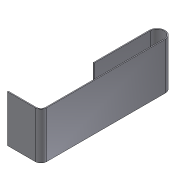
# Autodesk Inventor part: battery_tab_folded
Saved by Autodesk Inventor 2014 SP1 (Build 180222100, 222)
## iProperties
Created: 2013-03-29
Part Number: battery_tab_folded
Document SubType Name: Modeling
Designer: Robert Davis
Density: 7.85 g/cm^3
Material: Steel
Mass: 0.0909133 g
Surface Area: 2.37259 cm^2
Volume: 0.0115813 cm^3
Appearance: Steel
Author: Robert Davis
Autodesk Inventor part; units mm, degrees
ref_plane "YZ Plane" through (0, 0, 0) normal (1, 0, 0) x (0, 1, 0)
ref_plane "XZ Plane" through (0, 0, 0) normal (0, 1, 0) x (-1, 0, 0)
ref_plane "XY Plane" through (0, 0, 0) normal (0, 0, 1) x (1, 0, 0)
sketch "Sketch1" plane through (0, 0, 0) normal (0, 0, 1) x (1, 0, 0)
  line L0 (0, -3) -> (0, 3)
  line L1 (1.5, 3) -> (1.5, -9.7)
  line L2 (1, -10.2) -> (-2, -10.2)
  arc A0 (1.5, 3) -> (0, 3) centre (0.75, 3) ccw
  arc A1 (1, -10.2) -> (1.5, -9.7) centre (1, -9.7) ccw
  line L3 (-2, -10.3) -> (1, -10.3)
  arc A2 (1, -10.3) -> (1.6, -9.7) centre (1, -9.7) ccw
  line L4 (1.6, -9.7) -> (1.6, 3)
  arc A3 (1.6, 3) -> (-0.1, 3) centre (0.75, 3) ccw
  line L5 (-0.1, 3) -> (-0.1, -3)
  line L6 (0, -3) -> (-0.1, -3)
  line L7 (-2, -10.2) -> (-2, -10.3)
  point P0 (0, 0)
  point P1 (1.3536, -10.0536)
  dimension "d0" = 0.5
  dimension "d1" = 0.75
  dimension "d2" = 3
  dimension "d3" = 3
  dimension "d5" = 3
  dimension "d6" = 0.1
  dimension "d9" = 10.2
  constraints: 16 end point, 9 point on circle, 4 centre point, 4 tangent, 3 vertical, 2 horizontal, 1 midpoint, 4 other
  measures "d0" radius of A1
  measures "d1" radius of A0
  measures "d2" distance of L0.start point (0, 0)
  measures "d3" distance of L0.end point (0, 0)
  measures "d5" distance of L2.start L2.end
  measures "d6" distance of L2.end L3.start
  measures "d9" distance from line of point (0, 0) L2
extrude "Extrusion1" add sketch "Sketch1" along normal mid plane 5
body "Solid1"
